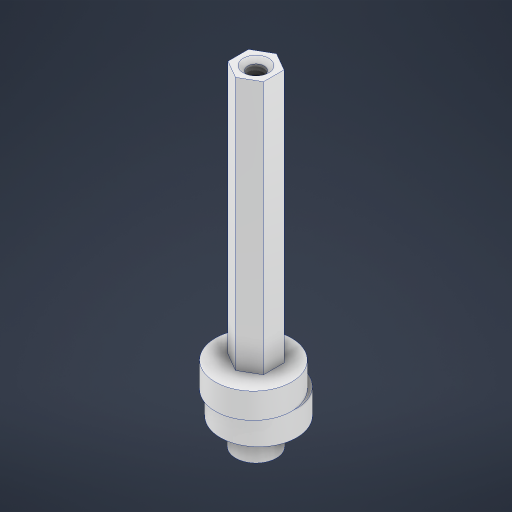
# Autodesk Inventor part: SHAFT_GB
Saved by Autodesk Inventor 2024.2 (Build 282272000, 272)
## iProperties
Created: 2026-01-03
Part Number: SHAFT_GB
Material: Aluminum 6061
Document SubType Name: Modeling
Designer: 4aida
Density: 2.7 g/cm^3
Appearance: Aluminum - Flat
Author: 4aida
Autodesk Inventor part; units mm, degrees
ref_plane "YZ Plane" through (0, 0, 0) normal (1, 0, 0) x (0, 1, 0)
ref_plane "XZ Plane" through (0, 0, 0) normal (0, 1, 0) x (-1, 0, 0)
ref_plane "XY Plane" through (0, 0, 0) normal (0, 0, 1) x (1, 0, 0)
sketch "Sketch1" plane through (0, 0, 0) normal (0, 1, 0) x (-1, 0, 0)
  circle A0 centre (0, 0.5) radius 7.5
  point P0 (0, 0)
  dimension "d0" = 0.5
  dimension "d1" = 15
  constraints: 1 centre point, 1 vertical alignment
  measures "d0" distance of point (0, 0) A0.centre
  measures "d1" diameter of A0
extrude "Extrusion1" add sketch "Sketch1" along normal blind 5
sketch "Sketch2" plane through (0, 0, 0.5) normal (0, -1, 0) x (1, 0, 0)
  circle A0 centre (0, -1) radius 7.5
  point P0 (0, -0.5)
  dimension "d4" = 0.5
  dimension "d5" = 15
  constraints: 1 centre point, 1 vertical alignment
  measures "d4" distance of A0.centre point (0, -0.5)
  measures "d5" diameter of A0
extrude "Extrusion2" add sketch "Sketch2" along normal blind 5
sketch "Sketch3" plane through (0, -5, -0.5) normal (0, -1, 0) x (1, 0, 0)
  circle A0 centre (0, 0.5) radius 4
  dimension "d14" = 8
  constraints: 2 coincident, 1 centre point
  measures "d14" diameter of A0
extrude "Extrusion3" add sketch "Sketch3" along normal blind 5
sketch "Sketch5" plane through (0, 5, 0.5) normal (0, 1, 0) x (1, 0, 0)
  line L0 (-3.5, -1.5207) -> (-3.5, 2.5207)
  line L1 (-3.5, 2.5207) -> (0, 4.5415)
  line L2 (0, 4.5415) -> (3.5, 2.5207)
  line L3 (3.5, 2.5207) -> (3.5, -1.5207)
  line L4 (3.5, -1.5207) -> (0, -3.5415)
  line L5 (0, -3.5415) -> (-3.5, -1.5207)
  point P0 (0, 0.5)
  point P1 (0, 0.5)
  point P2 (0, 0.5)
  dimension "d15" = 7
  constraints: 12 end point, 1 coincident, 1 vertical, 13 other
  measures "d15" distance between parallel lines of L0 L3
extrude "Extrusion5" add sketch "Sketch5" along normal blind 50
sketch "Sketch6" plane through (0, 55, 0.5) normal (0, 1, 0) x (1, 0, 0)
  point P0 (0, 0.5)
hole "Hole1" at (0, 55, 0) direction (0, -1, 0) diameter 3.242 depth 11.8 tip angle 118 countersink diameter 5 countersink angle 90 thread size "M4x0.7" class "6H" standard "ANSI Metric M Profile"
sketch "Sketch7" plane through (0, -10, 0) normal (0, -1, 0) x (1, 0, 0)
  point P0 (0, 0)
hole "Hole2" at (0, -10, 0) direction (0, 1, 0) diameter 3.242 depth 11.8 tip angle 118 countersink diameter 5 countersink angle 90 thread size "M4x0.7" class "6H" standard "ANSI Metric M Profile"
equation "\"d4\" = d0"
equation "\"d5\" = d1"
equation "\"d6\" = d2"
equation "\"d2\" = 5"
body "Solid1"
